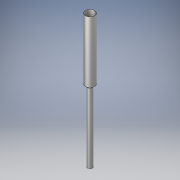
# Autodesk Inventor part: still pipe unmodified
Saved by Autodesk Inventor 2018 (Build 220112000, 112)
## iProperties
Created: 2019-01-14
Part Number: still pipe unmodified
Material: Stainless Steel AISI 304
Document SubType Name: Modeling
Designer: Admin
Density: 8 g/cm^3
Appearance: Chrome - Satin
Author: Admin
Autodesk Inventor part; units mm, degrees
ref_plane "YZ Plane" through (0, 0, 0) normal (1, 0, 0) x (0, 1, 0)
ref_plane "XZ Plane" through (0, 0, 0) normal (0, 1, 0) x (-1, 0, 0)
ref_plane "XY Plane" through (0, 0, 0) normal (0, 0, 1) x (1, 0, 0)
sketch "Sketch1" plane through (0, 0, 0) normal (0, 1, 0) x (-1, 0, 0)
  circle A0 centre (0, 0) radius 25.4635
  circle A1 centre (0, 0) radius 24.5237
  dimension "d0" = 50.927
  dimension "d1" = 0.9398
  constraints: 2 centre point, 2 coincident
  measures "d0" diameter of A0
  measures "d1" radial gap between concentric circles of A0 A1
extrude "Extrusion1" add sketch "Sketch1" against normal blind 332.5
sketch "Sketch2" plane through (0, -332.5, 0) normal (0, -1, 0) x (1, 0, 0)
  circle A0 centre (0, 0) radius 14.2875
  circle A1 centre (0, 0) radius 25.4635
  circle A2 centre (0, 0) radius 25.4635 projected
  dimension "d4" = 28.575
  constraints: 2 centre point, 2 coincident, 1 concentric
  measures "d4" diameter of A0
extrude "Extrusion2" add sketch "Sketch2" along normal blind 0.9398
sketch "Sketch3" plane through (0, -332.5, 0) normal (0, 1, 0) x (1, 0, 0)
  circle A0 centre (0, 0) radius 14.2875
  circle A1 centre (0, 0) radius 14.2875 projected
  circle A2 centre (0, 0) radius 13.3477
  dimension "d7" = 0.9398
  constraints: 2 centre point, 2 coincident, 1 concentric
  measures "d7" radial gap between concentric circles of A2 A0
extrude "Extrusion3" add sketch "Sketch3" against normal blind 11.811
sketch "Sketch4" plane through (0, -344.311, 0) normal (0, -1, 0) x (1, 0, 0)
  circle A0 centre (0, 0) radius 13.3477
  circle A1 centre (0, 0) radius 13.3477 projected
  circle A2 centre (0, 0) radius 12.4079
  dimension "d10" = 0.9398
  constraints: 2 centre point, 2 coincident, 1 concentric
  measures "d10" radial gap between concentric circles of A0 A2
extrude "Extrusion4" add sketch "Sketch4" along normal blind 381 and the other way blind 5.08
fillet "Fillet1" radius 3.175 1 edges at (-14.2875, -333.4398, 0)
fillet "Fillet2" radius 0.508 1 edges at (-13.3477, -344.311, 0)
body "Solid1"
